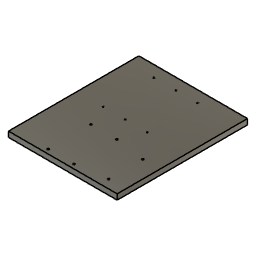
Wood Base v2 (Autodesk Fusion 360 design; units mm, degrees)
Autodesk Fusion 360 part; units mm, degrees
sketch "sketch 298" plane through (0, 0, 0) normal (0, 0, 1) x (1, 0, 0)
  circle A0 centre (191.7498, 150) radius 1.6
  circle A1 centre (110, 0) radius 2.25
  circle A2 centre (88.7502, 150) radius 1.6
  circle A3 centre (191.4838, 268) radius 1.6
  circle A4 centre (170.5, 100) radius 2.25
  circle A5 centre (241.25, 10) radius 2.25
  circle A6 centre (140.25, 150) radius 1.6
  circle A7 centre (241.25, 90) radius 2.25
  circle A8 centre (89.0162, 268) radius 1.6
  circle A9 centre (140.25, 268) radius 1.6
  circle A10 centre (170.5, 0) radius 2.25
  circle A11 centre (110, 100) radius 2.25
  line L0 (27.25, 294.8) -> (281.25, 294.8)
  line L1 (27.25, -10) -> (27.25, 294.8)
  line L2 (281.25, -10) -> (27.25, -10)
  line L3 (281.25, 294.8) -> (281.25, -10)
extrude "Extrude1" add sketch "sketch 298" against normal blind 12.7
